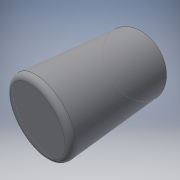
# Autodesk Inventor part: 3775
Saved by Autodesk Inventor 2019 (Build 230136000, 136)
## iProperties
Created: 2018-10-12
Part Number: 3775
Material: Generic
Document SubType Name: Modeling
Designer: Adhik
Density: 3.51389 g/cm^3
Appearance: Default
Mass: 366 g
Surface Area: 122.894 cm^2
Volume: 104.158 cm^3
Author: Adhik
Autodesk Inventor part; units mm, degrees
ref_plane "YZ Plane" through (0, 0, 0) normal (1, 0, 0) x (0, 1, 0)
ref_plane "XZ Plane" through (0, 0, 0) normal (0, 1, 0) x (-1, 0, 0)
ref_plane "XY Plane" through (0, 0, 0) normal (0, 0, 1) x (1, 0, 0)
sketch "Sketch1" plane through (0, 0, 0) normal (0, 0, 1) x (1, 0, 0)
  circle A0 centre (0, 0) radius 22.352
  dimension "d0" = 44.704
  constraints: 1 centre point, 1 coincident
  measures "d0" diameter of A0
extrude "Extrusion1" add sketch "Sketch1" along normal mid plane 66.548
fillet "Fillet1" radius 3.175 1 edges at (-22.352, 0, 33.274)
body "Solid1"
